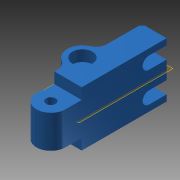
# Autodesk Inventor part: OfflineBowdenExtruderIdler
Saved by Autodesk Inventor 2015 SP1 (Build 190203100, 203)
## iProperties
Created: 2015-04-29
Part Number: OfflineBowdenExtruderIdler
Material: Generic
Document SubType Name: Modeling
Designer: Jack
Density: 1 g/cm^3
Appearance: Cyan
Author: Jack
Autodesk Inventor part; units mm, degrees
ref_plane "YZ Plane" through (0, 0, 0) normal (1, 0, 0) x (0, 1, 0)
ref_plane "XZ Plane" through (0, 0, 0) normal (0, 1, 0) x (-1, 0, 0)
ref_plane "XY Plane" through (0, 0, 0) normal (0, 0, 1) x (1, 0, 0)
sketch "Sketch1" plane through (0, 0, 0) normal (0, 0, 1) x (1, 0, 0)
  arc A0 (-4.75, 2.2361) -> (5.25, 0) centre (0, 0) ccw
  line L0 (5.25, 0) -> (5.25, 37)
  line L1 (5.25, 37) -> (-3.75, 37)
  arc A1 (-3.75, 20.9943) -> (-4.75, 10.0514) centre (-4, 15.5) ccw
  line L2 (-3.75, 37) -> (-3.75, 20.9943)
  line L3 (-4.75, 10.0514) -> (-4.75, 2.2361)
  dimension "d0" = 10.5
  dimension "d1" = 37
  dimension "d3" = 4
  dimension "d4" = 15.5
  dimension "d5" = 11
  dimension "d22" = 10
  dimension "d23" = 9
  constraints: 8 end point, 4 point on circle, 2 centre point, 2 vertical, 1 coincident, 1 perpendicular, 1 tangent
  measures "d0" diameter of A0
  measures "d1" distance from line of point (0, 0) L1
  measures "d3" horizontal distance of point (0, 0) A1.centre
  measures "d4" vertical distance of point (0, 0) A1.centre
  measures "d5" diameter of A1
  measures "d22" distance between parallel lines of L0 L3
  measures "d23" distance between parallel lines of L0 L2
extrude "Extrusion1" add sketch "Sketch1" along normal blind 20
sketch "Sketch2" plane through (0, 0, 20) normal (0, 0, 1) x (1, 0, 0)
  arc A0 (-4.75, 2.2361) -> (5.25, 0) centre (0, 0) ccw projected
  line L0 (5.25, 0) -> (5.25, 37) projected
  line L1 (-4.75, 10.0514) -> (-4.75, 2.2361) projected
  line L2 (-4.75, 6) -> (5.25, 6)
  dimension "d9" = 6
  constraints: 2 end point, 2 point on line, 1 perpendicular
  measures "d9" distance from line of A0.centre L2
extrude "Extrusion2" cut sketch "Sketch2" against normal blind 4
sketch "Sketch3" plane through (0, 0, 0) normal (0, 0, -1) x (-1, 0, 0)
  arc A0 (-5.25, 0) -> (4.75, 2.2361) centre (0, 0) ccw projected
  line L0 (4.75, 2.2361) -> (4.75, 10.0514) projected
  line L1 (-5.25, 37) -> (-5.25, 0) projected
  line L2 (4.75, 6) -> (-5.25, 6) projected
extrude "Extrusion3" cut sketch "Sketch3" against normal blind 4
fillet "Fillet1" radius 4 2 edges at (-3.75, 20.9943, 10) (-4.75, 10.0514, 10)
sketch "Sketch4" plane through (0, 0, 16) normal (0, 0, 1) x (1, 0, 0)
  arc A0 (-4.75, 2.2361) -> (5.25, 0) centre (0, 0) ccw projected
hole "Hole1" at (0, 0, 16) direction (0, 0, -1) diameter 3.5 end through all
sketch "Sketch5" plane through (5.25, 37, 20) normal (1, 0, 0) x (0, 0, -1)
  line L0 (20, 0) -> (20, -31) projected
  line L1 (20, 0) -> (0, 0) projected
  arc A0 (2.25, -6.5) -> (6.75, -6.5) centre (4.5, -6.5) ccw
  arc A1 (13.25, -6.5) -> (17.75, -6.5) centre (15.5, -6.5) ccw
  line L2 (6.75, -6.5) -> (6.75, 0)
  line L3 (2.25, -6.5) -> (2.25, 0)
  line L4 (13.25, -6.5) -> (13.25, 0)
  line L5 (17.75, -6.5) -> (17.75, 0)
  point P0 (20, -37)
  dimension "d24" = 4.5
  dimension "d25" = 6.5
  dimension "d26" = 11
  dimension "d27" = 4.5
  constraints: 8 end point, 4 perpendicular, 4 point on circle, 4 point on line, 4 tangent, 2 centre point, 1 equal radius, 1 horizontal alignment
  measures "d24" diameter of A0
  measures "d25" distance from line of L1 A0.centre
  measures "d26" distance of A1.centre A0.centre
  measures "d27" distance from line of L0 A1.centre
extrude "Extrusion4" cut sketch "Sketch5" against normal up to next
chamfer "Chamfer1" distance 1 angle 45 3 edges at (-3.75, 37, 18.875) (-3.75, 37, 10) (-3.75, 37, 1.125)
ref_plane "Work Plane1" through (0, 0, 10) normal (0, 0, 1) x (1, 0, 0)
sketch "Sketch6" plane through (0, 0, 10) normal (0, 0, 1) x (1, 0, 0)
  arc A0 (-6.1711, 20.5534) -> (-6.75, 10.7369) centre (-4, 15.5) ccw projected
  circle A1 centre (-4, 15.5) radius 7
  point P0 (0, 0)
  dimension "d34" = 14
  constraints: 1 centre point, 1 coincident
  measures "d34" diameter of A1
extrude "Extrusion5" cut sketch "Sketch6" along normal mid plane 6
sketch "Sketch7" plane through (0, 0, 20) normal (0, 0, 1) x (1, 0, 0)
  arc A0 (-6.1711, 20.5534) -> (-6.75, 10.7369) centre (-4, 15.5) ccw projected
  point P0 (0, 0)
hole "Hole2" at (-4, 15.5, 20) direction (0, 0, -1) diameter 3.5 end through all counterbore diameter 7.4 counterbore depth 4
sketch "Sketch8" plane through (0, 0, 7) normal (0, 0, 1) x (1, 0, 0)
  circle A0 centre (-4, 15.5) radius 1.75 projected
  arc A1 (-6.1711, 20.5534) -> (-6.75, 10.7369) centre (-4, 15.5) ccw projected
  circle A2 centre (-4, 15.5) radius 2.5
  point P0 (0, 0)
  dimension "d44" = 5
  constraints: 1 centre point, 1 coincident
  measures "d44" diameter of A2
extrude "Extrusion6" add sketch "Sketch8" along normal blind 0.5
sketch "Sketch9" plane through (0, 0, 13) normal (0, 0, -1) x (-1, 0, 0)
  circle A0 centre (4, 15.5) radius 1.75 projected
  arc A1 (4.1435, 22.4985) -> (4.9651, 8.5669) centre (4, 15.5) ccw projected
  circle A2 centre (4, 15.5) radius 2.5
  point P0 (0, 0)
  dimension "d47" = 5
  constraints: 1 centre point, 1 coincident
  measures "d47" diameter of A2
extrude "Extrusion7" add sketch "Sketch9" along normal blind 0.5
chamfer "Chamfer2" distance 0.5 angle 45 2 edges at (-1.5, 15.5, 13) (-6.5, 15.5, 7)
sketch "Sketch10" plane through (0, 0, 0) normal (0, 0, -1) x (-1, 0, 0)
  circle A0 centre (4, 15.5) radius 1.75 projected
  arc A1 (6.75, 10.7369) -> (4.75, 7.2728) centre (8.75, 7.2728) ccw projected
  arc A2 (6.75, 10.7369) -> (6.1711, 20.5534) centre (4, 15.5) ccw projected
  arc A3 (3.75, 24.2285) -> (6.1711, 20.5534) centre (7.75, 24.2285) ccw projected
  arc A4 (3.75, 24.2285) -> (6.1711, 20.5534) centre (7.75, 24.2285) ccw projected
  arc A5 (5.3971, 20.9938) -> (5.5701, 9.6994) centre (15.5, 15.5) ccw
  point P0 (0, 0)
  dimension "d53" = 11.5
  dimension "d54" = 11.5
  constraints: 5 point on circle, 1 centre point, 1 horizontal alignment
  measures "d53" radius of A5
  measures "d54" distance of A0.centre A5.centre
extrude "Extrusion8" cut sketch "Sketch10" against normal blind 2.5 contours A0 A5 | A0 A5 A3 A2 A1 picked at (4.5932, 15.5)
sketch "Sketch11" plane through (0, 0, 2.5) normal (0, 0, -1) x (-1, 0, 0)
  arc A0 (6.75, 10.7369) -> (6.1711, 20.5534) centre (4, 15.5) ccw projected
  line L0 (8.2724, 15.5) -> (6.1362, 11.8)
  line L1 (6.1362, 11.8) -> (1.8638, 11.8)
  line L2 (1.8638, 11.8) -> (-0.2724, 15.5)
  line L3 (-0.2724, 15.5) -> (1.8638, 19.2)
  line L4 (1.8638, 19.2) -> (6.1362, 19.2)
  line L5 (6.1362, 19.2) -> (8.2724, 15.5)
  point P0 (0, 0)
  dimension "d57" = 7.4
  constraints: 12 end point, 1 coincident, 1 horizontal, 13 other
  measures "d57" distance between parallel lines of L4 L1
extrude "Extrusion9" cut sketch "Sketch11" against normal blind 3.5 and the other way blind 2.5
sketch "Sketch12" plane through (0, 0, 20) normal (0, 0, 1) x (1, 0, 0)
  line L0 (5.25, 6) -> (5.25, 37) projected
  line L1 (5.25, 30.5) -> (5.25, 28.25) projected
  line L2 (5.25, 30.5) -> (5.25, 28.25) projected
  line L3 (5.25, 37) -> (5.25, 30.5) projected
  arc A0 (5.25, 32.0731) -> (5.25, 28.8731) centre (6.45, 30.4731) ccw
  line L4 (-44.8411, 30.5865) -> (13.9588, 30.4731)
  point P0 (0, 0)
  point P1 (-44.8411, 30.5865)
  point P2 (13.9588, 30.4731)
  dimension "d62" = 2
  dimension "d63" = 1.2
  constraints: 2 point on circle, 2 point on line, 1 centre point, 1 horizontal alignment, 5 other
  measures "d62" radius of A0
  measures "d63" distance from line of L0 A0.centre
extrude "Extrusion10" cut sketch "Sketch12" against normal up to surface (20 mm away)
body "Solid1"
